Support Bobine 2 (Autodesk Fusion 360 design; units mm, degrees)
Autodesk Fusion 360 part; units mm, degrees
sketch "Sketch1" plane through (0, 0, 0) normal (0, 0, 1) x (1, 0, 0)
  circle A0 centre (0, 0) radius 14
  circle A1 centre (0, 0) radius 16
  circle A2 centre (0, 0) radius 6.5
  dimension "d1" = 28
  dimension "d2" = 2
  dimension "d10" = 13
  constraint coincident A0.centre A1.centre
  measures "d1" diameter of A0
  measures "d10" diameter of A2
extrude "Extrude4" add sketch "Sketch1" along normal blind 10 contours A0
sketch "Sketch2" plane through (0, 0, 10) normal (0, 0, 1) x (-1, 0, 0)
  circle A0 centre (0, 0) radius 14
  circle A1 centre (0, 0) radius 11.1
  circle A2 centre (0, 0) radius 6.5
  circle A3 centre (0, 0) radius 6.5
  circle A4 centre (0, 0) radius 14
  circle A5 centre (0, 0) radius 6.5
  circle A6 centre (0, 0) radius 14
  dimension "d7" = 22.2
  constraint coincident A0.centre A1.centre
  measures "d7" diameter of A1
extrude "Extrude5" cut sketch "Sketch2" against normal blind 7 contours A1
extrude "Extrude6" add sketch "Sketch1" along normal blind 2 contours A1
